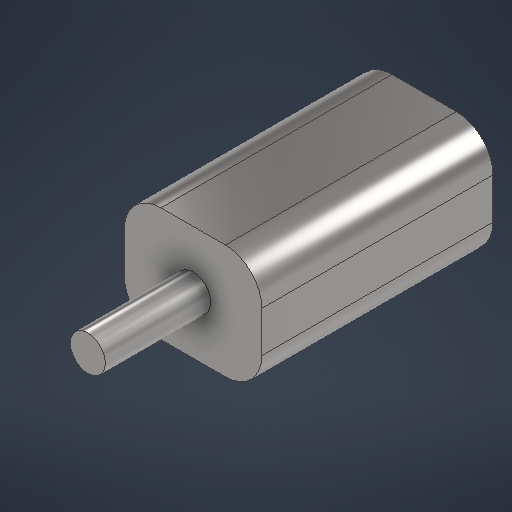
# Autodesk Inventor part: OGGearMotor
Saved by Autodesk Inventor 2027 (Build 310192060, 192F)
## iProperties
Created: 2026-07-12
Part Number: OGGearMotor
Material: Steel, Carbon
Document SubType Name: Modeling
Designer: machnach0
Density: 7.85 g/cm^3
Appearance: Semi-Polished
Author: machnach0
Autodesk Inventor part; units mm, degrees
ref_plane "YZ Plane" through (0, 0, 0) normal (1, 0, 0) x (0, 1, 0)
ref_plane "XZ Plane" through (0, 0, 0) normal (0, 1, 0) x (-1, 0, 0)
ref_plane "XY Plane" through (0, 0, 0) normal (0, 0, 1) x (1, 0, 0)
sketch "Sketch1" plane through (0, 0, 0) normal (0, 0, 1) x (1, 0, 0)
  line L0 (0, 0) -> (11.938, 0)
  line L1 (11.938, 0) -> (11.938, 9.906)
  line L2 (11.938, 9.906) -> (0, 9.906)
  line L3 (0, 9.906) -> (0, 0)
  circle A0 centre (5.969, 4.953) radius 1.524
  point P0 (0, 4.953)
  point P1 (5.969, 9.906)
  dimension "d0" = 11.938
  dimension "d1" = 9.906
  dimension "d2" = 3.048
  constraints: 8 end point, 2 midpoint, 2 parallel, 1 centre point, 1 horizontal, 1 horizontal alignment, 1 perpendicular, 1 vertical alignment
  measures "d0" distance of L1.end L2.end
  measures "d1" distance of L0.end L1.end
  measures "d2" diameter of A0
extrude "Extrusion1" add sketch "Sketch1" along normal blind 20.066 contours L3 L2 L1 L0 | A0
extrude "Extrusion2" add sketch "Sketch1" along normal blind 29.21 contours A0
fillet "Fillet1" radius 3.175 4 edges at (11.938, 9.906, 10.033) (11.938, 0, 10.033) (0, 9.906, 10.033) (0, 0, 10.033)
body "Solid1"
